Autodesk Fusion 360 part; units mm, degrees
(part 2 of 2)
extrude "Extrude1''''''" add sketch "Sketch15" along normal mid plane 2 separate body makes body 11 in component "Component'''''''"
sketch "Sketch16" plane through (0, -1, 0) normal (0, -1, 0) x (1, 0, 0)
  circle A0 centre (384.4482, -130.0025) radius 1.5
  line L0 (373.5366, -60.8681) -> (354.4293, -66.7768)
  line L1 (354.4293, -66.7768) -> (377.8488, -142.5104)
  line L2 (377.8488, -142.5104) -> (396.9561, -136.6018)
  line L3 (396.9561, -136.6018) -> (373.5366, -60.8681)
  circle A1 centre (384.4482, -130.0025) radius 20
  dimension "d131" = 40
  constraint concentric A0 A1
  measures "d131" diameter of A1
extrude "Extrude5" add sketch "Sketch16" along normal blind 15 separate body contours L1 L2 L3 A1 | L1 L2 L3 A1 makes body 12
move_body "Move2" bodies 10 to x (1, 0, 0) y (0, 1, 0) z (0, 0, 1) at (0, -20, 0) in component "Component''''''"
move_body "Move3" bodies 10 to x (1, 0, 0) y (0, 1, 0) z (0, 0, 1) at (0, 20, 0) in component "Component''''''"
move_face "OffsetFaces1" offset -10 2 faces at (109.5307, 25, -7.121) (62.8557, 25, -78.3124) on bodies 3 in component "Component'"
sketch "Sketch18" plane through (0, -25, 0) normal (0, -1, 0) x (1, 0, 0)
  line L0 (-154.4605, -86.8115) -> (-154.4605, -54.8376)
  arc A0 (-133.5015, -50.3854) -> (-154.4605, -54.8376) centre (-125.8317, -138.0506) ccw
  line L1 (-133.5015, -50.3854) -> (-100.5795, -47.5051)
  arc A1 (-100.5795, -47.5051) -> (-65.5572, -34.7581) centre (-106.8547, 24.2209) ccw
  line L2 (-65.5572, -34.7581) -> (-36.1822, -14.1895)
  line L3 (-36.1822, -14.1895) -> (-35.2306, -14.4872)
  line L4 (-35.2306, -14.4872) -> (-33.1659, -15.0291)
  line L5 (-33.1659, -15.0291) -> (-31.1204, -15.4888)
  line L6 (-31.1204, -15.4888) -> (-29.0261, -15.868)
  line L7 (-29.0261, -15.868) -> (-25.4452, -16.3609)
  line L8 (-25.4452, -16.3609) -> (-23.9353, -16.5361)
  line L9 (-23.9353, -16.5361) -> (-23.9353, -4.4556)
  line L10 (-23.9353, -4.4556) -> (-27.138, -4.0148)
  line L11 (-27.138, -4.0148) -> (-28.7346, -3.7257)
  line L12 (-28.7346, -3.7257) -> (-30.3263, -3.3679)
  line L13 (-30.3263, -3.3679) -> (-31.914, -2.9513)
  line L14 (-31.914, -2.9513) -> (-33.4961, -2.4562)
  line L15 (-33.4961, -2.4562) -> (-34.7442, -1.8366)
  line L16 (-34.7442, -1.8366) -> (-35.3615, -1.3596)
  line L17 (-35.3615, -1.3596) -> (-35.9566, -0.7068)
  line L18 (-35.9566, -0.7068) -> (-36.2502, -0.2525)
  line L19 (-36.2502, -0.2525) -> (-36.3957, 0.0633)
  line L20 (-36.3957, 0.0633) -> (-36.4605, 0.265)
  line L21 (-36.4605, 0.265) -> (-72.4401, -24.9282)
  arc A2 (-101.6254, -35.5508) -> (-72.4401, -24.9282) centre (-106.8547, 24.2209) ccw
  line L22 (-101.6254, -35.5508) -> (-134.5473, -38.4311)
  arc A3 (-134.5473, -38.4311) -> (-159.8637, -44.0196) centre (-125.8317, -138.0506) ccw
  arc A4 (-159.8637, -44.0196) -> (-166.4605, -53.4227) centre (-156.4605, -53.4227) ccw
  line L23 (-166.4605, -53.4227) -> (-166.4605, -88.4227)
  arc A5 (-166.4605, -88.4227) -> (-158.5986, -98.1914) centre (-156.4605, -88.4227) ccw
  spline S0 degree 3 poles (-158.5986, -98.1914) (-117.7698, -107.1276) (-84.5053, -111.2062) (-23.1255, -114.8448) (17.9002, -115.6029) (132.9422, -111.3091) (193.3206, -107.1118) (317.2109, -92.6975) (374.7187, -81.9546) (426.1581, -67.9976) knots 0 0 0 0 12.538582 12.538582 23.298988 23.298988 33.005579 33.005579 44.857348 44.857348 44.857348 44.857348
  arc A6 (426.1581, -67.9976) -> (433.5395, -58.3466) centre (423.5395, -58.3466) ccw
  line L24 (433.5395, -58.3466) -> (433.5395, -46.3466)
  line L25 (433.5395, -46.3466) -> (369.1135, -46.3466)
  spline S1 degree 3 poles (369.1135, -46.3466) (368.4873, -46.3489) (367.7595, -46.351) (366.4616, -46.3521) (365.7936, -46.3512) (365.1135, -46.3466) knots 0 0 0 0 0.187855 0.187855 0.377645 0.377645 0.377645 0.377645
  line L26 (365.1135, -46.3466) -> (365.1135, -36.3466)
  spline S2 degree 3 poles (365.1135, -36.3466) (322.4324, -36.2198) (274.1497, -35.2585) (209.4342, -29.8358) (172.1032, -25.0618) (125.1135, -10.3466) knots 0 0 0 0 12.804404 12.804404 22.769958 22.769958 22.769958 22.769958
  line L27 (125.1135, -10.3466) -> (122.8282, -9.6314)
  line L28 (122.8282, -9.6314) -> (121.2454, -9.1461)
  line L29 (121.2454, -9.1461) -> (119.6632, -8.651)
  line L30 (119.6632, -8.651) -> (118.0804, -8.1657)
  line L31 (118.0804, -8.1657) -> (114.9147, -7.1951)
  line L32 (114.9147, -7.1951) -> (111.747, -6.254)
  line L33 (111.747, -6.254) -> (108.5786, -5.3226)
  line L34 (108.5786, -5.3226) -> (108.2665, -5.2318)
  line L35 (108.2665, -5.2318) -> (108.2665, -9.7863)
  line L36 (108.2665, -9.7863) -> (105.0405, -9.679)
  line L37 (105.0405, -9.679) -> (101.8144, -9.5717)
  line L38 (101.8144, -9.5717) -> (101.8144, -21.5784)
  line L39 (101.8144, -21.5784) -> (104.6416, -21.6724)
  line L40 (104.6416, -21.6724) -> (111.0937, -21.887)
  line L41 (111.0937, -21.887) -> (114.3197, -21.9943)
  line L42 (114.3197, -21.9943) -> (122.3848, -22.2625)
  line L43 (122.3848, -22.2625) -> (123.2114, -22.29)
  spline S3 degree 3 poles (123.2114, -22.29) (133.5497, -25.285) (143.6571, -28.0575) (153.5395, -30.6156) knots -26.624685 -26.624685 -26.624685 -26.624685 -23.3972 -23.3972 -23.3972 -23.3972
  line L44 (153.5395, -30.6156) -> (153.5395, -91.8115)
  line L45 (153.5395, -91.8115) -> (-131.4605, -91.8115)
  line L46 (-131.4605, -91.8115) -> (-131.4605, -86.8115)
  line L47 (-131.4605, -86.8115) -> (-154.4605, -86.8115)
move_body "Move4" bodies 10 to x (1, 0, 0) y (0, 1, 0) z (0, 0, 1) at (0, -29.9, 0) in component "Component''''''"
move_face "MoveFace1" to x (1, 0, 0) y (0, 1, 0) z (0, 0, 1) at (0, 30.8, 0) 1 faces at (18.5022, -141.2333, -195.7508) on bodies 10 in component "Component''''''"
sketch "Sketch19" plane through (0.2272, -147.9, -0.2202) normal (0, -1, 0) x (1, 0, 0)
  circle A0 centre (-11.6877, -194.0352) radius 30
  line L0 (-54.0775, -241.7318) -> (180.0573, -241.7318)
  line L1 (180.0573, -241.7318) -> (180.0573, -333.6288)
  line L2 (180.0573, -333.6288) -> (-54.0775, -333.6288)
  line L3 (-54.0775, -333.6288) -> (-54.0775, -241.7318)
  circle A1 centre (128.0273, -293.086) radius 30
  circle A2 centre (56.4017, -293.086) radius 30
  circle A3 centre (-6.7775, -293.086) radius 20
  line L4 (128.0273, -293.086) -> (128.0273, -323.086) construction
  line L5 (56.4017, -293.086) -> (56.4017, -323.086) construction
  line L6 (-6.7775, -293.086) -> (-6.7775, -313.086) construction
  dimension "d153" = 60
  dimension "d154" = 60
  dimension "d155" = 40
  constraint horizontal L0
  constraint vertical L1
  constraint horizontal L2
  constraint vertical L3
  constraint horizontal A1.centre A2.centre
  constraint horizontal A2.centre A3.centre
  constraint coincident A1.centre L4.start
  constraint coincident A1 L4.end
  constraint perpendicular L0 L4
  constraint coincident A2.centre L5.start
  constraint coincident A2 L5.end
  constraint parallel L4 L5
  constraint coincident A3.centre L6.start
  constraint coincident A3 L6.end
  constraint perpendicular L0 L6
  measures "d153" diameter of A1
  measures "d154" diameter of A2
  measures "d155" diameter of A3
component "Component" placed x (1, 0, 0) y (0, 1, 0) z (0, 0, 1) at (0, 0, 0)
component "Component'" placed x (1, 0, 0) y (0, 1, 0) z (0, 0, 1) at (0, -10, 0)
component "Component''" placed x (1, 0, 0) y (0, 1, 0) z (0, 0, 1) at (0, 0, 0)
component "Component'" placed x (1, 0, 0) y (0, 1, 0) z (0, 0, 1) at (0, -70, 0)
component "Component'''" placed x (1, 0, 0) y (0, 1, 0) z (0, 0, 1) at (0, 0, 0)
component "Component''''" placed x (1, 0, 0) y (0, 1, 0) z (0, 0, 1) at (0, 0, 0)
component "Component'''''" placed x (1, 0, 0) y (0, 1, 0) z (0, 0, 1) at (0, 0, 0)
component "Component''''''" placed x (1, 0, 0) y (0, 1, 0) z (0, 0, 1) at (0, 0, 0)
component "Component''''''" placed x (1, 0, 0) y (0, 1, 0) z (0, 0, 1) at (0, 255, 0)
component "Component'''''''" placed x (1, 0, 0) y (0, 1, 0) z (0, 0, 1) at (0, 0, 0)
